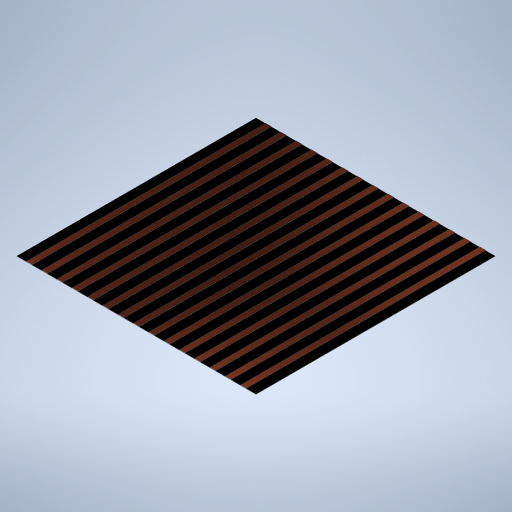
# Autodesk Inventor part: Sensor Grid Rows-Collumns
Saved by Autodesk Inventor 2023 (Build 270158000, 158)
## iProperties
Created: 2022-11-30
Part Number: Sensor Grid Rows-Collumns
Material: Generic
Document SubType Name: Modeling
Designer: dylan
Density: 1 g/cm^3
Appearance: Default
Author: dylan
Autodesk Inventor part; units mm, degrees
ref_plane "YZ Plane" through (0, 0, 0) normal (1, 0, 0) x (0, 1, 0)
ref_plane "XZ Plane" through (0, 0, 0) normal (0, 1, 0) x (-1, 0, 0)
ref_plane "XY Plane" through (0, 0, 0) normal (0, 0, 1) x (1, 0, 0)
sketch "Sketch1" plane through (0, 0, 0) normal (0, 1, 0) x (-1, 0, 0)
  line L0 (0, 0) -> (800, 0)
  line L1 (800, 0) -> (800, -800)
  line L2 (800, -800) -> (0, -800)
  line L3 (0, -800) -> (0, 0)
  line L4 (0, 0) -> (32.14, 0)
  line L5 (32.14, 0) -> (32.14, -800)
  line L6 (32.14, -800) -> (0, -800)
  line L7 (0, -800) -> (0, 0)
  line L8 (32.14, 0) -> (51.19, 0)
  line L9 (51.19, 0) -> (51.19, -800)
  line L10 (51.19, -800) -> (32.14, -800)
  line L11 (32.14, -800) -> (32.14, 0)
  line L12 (51.19, 0) -> (83.33, 0)
  line L13 (83.33, 0) -> (83.33, -800)
  line L14 (83.33, -800) -> (51.19, -800)
  line L15 (51.19, -800) -> (51.19, 0)
  line L16 (83.33, 0) -> (102.38, 0)
  line L17 (102.38, 0) -> (102.38, -800)
  line L18 (102.38, -800) -> (83.33, -800)
  line L19 (83.33, -800) -> (83.33, 0)
  line L20 (102.38, 0) -> (134.52, 0)
  line L21 (134.52, 0) -> (134.52, -800)
  line L22 (134.52, -800) -> (102.38, -800)
  line L23 (102.38, -800) -> (102.38, 0)
  line L24 (134.52, 0) -> (153.57, 0)
  line L25 (153.57, 0) -> (153.57, -800)
  line L26 (153.57, -800) -> (134.52, -800)
  line L27 (134.52, -800) -> (134.52, 0)
  line L28 (153.57, 0) -> (185.71, 0)
  line L29 (185.71, 0) -> (185.71, -800)
  line L30 (185.71, -800) -> (153.57, -800)
  line L31 (153.57, -800) -> (153.57, 0)
  line L32 (185.71, 0) -> (204.76, 0)
  line L33 (204.76, 0) -> (204.76, -800)
  line L34 (204.76, -800) -> (185.71, -800)
  line L35 (185.71, -800) -> (185.71, 0)
  line L36 (204.76, 0) -> (236.9, 0)
  line L37 (236.9, 0) -> (236.9, -800)
  line L38 (236.9, -800) -> (204.76, -800)
  line L39 (204.76, -800) -> (204.76, 0)
  line L40 (236.9, 0) -> (255.95, 0)
  line L41 (255.95, 0) -> (255.95, -800)
  line L42 (255.95, -800) -> (236.9, -800)
  line L43 (236.9, -800) -> (236.9, 0)
  line L44 (255.95, 0) -> (288.09, 0)
  line L45 (288.09, 0) -> (288.09, -800)
  line L46 (288.09, -800) -> (255.95, -800)
  line L47 (255.95, -800) -> (255.95, 0)
  line L48 (288.09, 0) -> (307.14, 0)
  line L49 (307.14, 0) -> (307.14, -800)
  line L50 (307.14, -800) -> (288.09, -800)
  line L51 (288.09, -800) -> (288.09, 0)
  line L52 (307.14, 0) -> (339.28, 0)
  line L53 (339.28, 0) -> (339.28, -800)
  line L54 (339.28, -800) -> (307.14, -800)
  line L55 (307.14, -800) -> (307.14, 0)
  line L56 (339.28, 0) -> (358.33, 0)
  line L57 (358.33, 0) -> (358.33, -800)
  line L58 (358.33, -800) -> (339.28, -800)
  line L59 (339.28, -800) -> (339.28, 0)
  line L60 (358.33, 0) -> (390.47, 0)
  line L61 (390.47, 0) -> (390.47, -800)
  line L62 (390.47, -800) -> (358.33, -800)
  line L63 (358.33, -800) -> (358.33, 0)
  line L64 (390.47, 0) -> (409.52, 0)
  line L65 (409.52, 0) -> (409.52, -800)
  line L66 (409.52, -800) -> (390.47, -800)
  line L67 (390.47, -800) -> (390.47, 0)
  line L68 (409.52, 0) -> (441.66, 0)
  line L69 (441.66, 0) -> (441.66, -800)
  line L70 (441.66, -800) -> (409.52, -800)
  line L71 (409.52, -800) -> (409.52, 0)
  line L72 (441.66, 0) -> (460.71, 0)
  line L73 (460.71, 0) -> (460.71, -800)
  line L74 (460.71, -800) -> (441.66, -800)
  line L75 (441.66, -800) -> (441.66, 0)
  line L76 (460.71, 0) -> (492.85, 0)
  line L77 (492.85, 0) -> (492.85, -800)
  line L78 (492.85, -800) -> (460.71, -800)
  line L79 (460.71, -800) -> (460.71, 0)
  line L80 (492.85, 0) -> (511.9, 0)
  line L81 (511.9, 0) -> (511.9, -800)
  line L82 (511.9, -800) -> (492.85, -800)
  line L83 (492.85, -800) -> (492.85, 0)
  line L84 (511.9, 0) -> (544.04, 0)
  line L85 (544.04, 0) -> (544.04, -800)
  line L86 (544.04, -800) -> (511.9, -800)
  line L87 (511.9, -800) -> (511.9, 0)
  line L88 (544.04, 0) -> (563.09, 0)
  line L89 (563.09, 0) -> (563.09, -800)
  line L90 (563.09, -800) -> (544.04, -800)
  line L91 (544.04, -800) -> (544.04, 0)
  line L92 (563.09, 0) -> (595.23, 0)
  line L93 (595.23, 0) -> (595.23, -800)
  line L94 (595.23, -800) -> (563.09, -800)
  line L95 (563.09, -800) -> (563.09, 0)
  line L96 (595.23, 0) -> (614.28, 0)
  line L97 (614.28, 0) -> (614.28, -800)
  line L98 (614.28, -800) -> (595.23, -800)
  line L99 (595.23, -800) -> (595.23, 0)
  line L100 (614.28, 0) -> (646.42, 0)
  line L101 (646.42, 0) -> (646.42, -800)
  line L102 (646.42, -800) -> (614.28, -800)
  line L103 (614.28, -800) -> (614.28, 0)
  line L104 (646.42, 0) -> (665.47, 0)
  line L105 (665.47, 0) -> (665.47, -800)
  line L106 (665.47, -800) -> (646.42, -800)
  line L107 (646.42, -800) -> (646.42, 0)
  line L108 (665.47, 0) -> (697.61, 0)
  line L109 (697.61, 0) -> (697.61, -800)
  line L110 (697.61, -800) -> (665.47, -800)
  line L111 (665.47, -800) -> (665.47, 0)
  line L112 (697.61, 0) -> (716.66, 0)
  line L113 (716.66, 0) -> (716.66, -800)
  line L114 (716.66, -800) -> (697.61, -800)
  line L115 (697.61, -800) -> (697.61, 0)
  line L116 (716.66, 0) -> (748.8, 0)
  line L117 (748.8, 0) -> (748.8, -800)
  line L118 (748.8, -800) -> (716.66, -800)
  line L119 (716.66, -800) -> (716.66, 0)
  line L120 (748.8, 0) -> (767.85, 0)
  line L121 (767.85, 0) -> (767.85, -800)
  line L122 (767.85, -800) -> (748.8, -800)
  line L123 (748.8, -800) -> (748.8, 0)
  dimension "d0" = 800
  dimension "d1" = 800
  dimension "d2" = 32.14
  dimension "d4" = 19.05
  dimension "d6" = 32.14
  dimension "d7" = 19.05
  dimension "d8" = 32.14
  dimension "d9" = 19.05
  dimension "d10" = 32.14
  dimension "d11" = 19.05
  dimension "d12" = 32.14
  dimension "d13" = 19.05
  dimension "d14" = 32.14
  dimension "d15" = 19.05
  dimension "d16" = 32.14
  dimension "d17" = 19.05
  dimension "d18" = 32.14
  dimension "d19" = 19.05
  dimension "d20" = 32.14
  dimension "d21" = 19.05
  dimension "d22" = 32.14
  dimension "d23" = 19.05
  dimension "d24" = 32.14
  dimension "d25" = 19.05
  dimension "d26" = 32.14
  dimension "d27" = 19.05
  dimension "d28" = 32.14
  dimension "d29" = 19.05
  dimension "d30" = 32.14
  dimension "d31" = 19.05
  dimension "d32" = 32.14
  dimension "d33" = 19.05
  constraints: 244 end point, 61 parallel, 30 horizontal, 30 perpendicular, 1 vertical, 6 other
  measures "d0" distance of L1.end L3.start
  measures "d1" distance of L1.start L1.end
  measures "d2" distance of L5.end L6.end
  measures "d4" distance of L9.end L10.end
  measures "d6" distance of L13.end L14.end
  measures "d7" distance of L17.end L18.end
  measures "d8" distance of L21.end L22.end
  measures "d9" distance of L25.end L26.end
  measures "d10" distance of L29.end L30.end
  measures "d11" distance of L33.end L34.end
  measures "d12" distance of L37.end L38.end
  measures "d13" distance of L41.end L42.end
  measures "d14" distance of L45.end L46.end
  measures "d15" distance of L49.end L50.end
  measures "d16" distance of L53.end L54.end
  measures "d17" distance of L57.end L58.end
  measures "d18" distance of L61.end L62.end
  measures "d19" distance of L65.end L66.end
  measures "d20" distance of L69.end L70.end
  measures "d21" distance of L73.end L74.end
  measures "d22" distance of L77.end L78.end
  measures "d23" distance of L81.end L82.end
  measures "d24" distance of L85.end L86.end
  measures "d25" distance of L89.end L90.end
  measures "d26" distance of L93.end L94.end
  measures "d27" distance of L97.end L98.end
  measures "d28" distance of L101.end L102.end
  measures "d29" distance of L105.end L106.end
  measures "d30" distance of L109.end L110.end
  measures "d31" distance of L113.end L114.end
  measures "d32" distance of L117.end L118.end
  measures "d33" distance of L121.end L122.end
extrude "Extrusion1" add sketch "Sketch1" along normal blind 1 contours L0 L5 L2 L3 | L0 L13 L2 L9 | L0 L21 L2 L17 | L0 L29 L2 L25 | L0 L37 L2 L33 | L0 L45 L2 L41 | L0 L53 L2 L49 | L0 L61 L2 L57 | L0 L69 L2 L65 | L0 L77 L2 L73 | L0 L85 L2 L81 | L0 L93 L2 L89 | L0 L101 L2 L97 | L0 L109 L2 L105 | L0 L117 L2 L113 | L0 L1 L2 L121
extrude "Extrusion2" add sketch "Sketch1" along normal blind 2 contours L0 L9 L2 L5 | L0 L17 L2 L13 | L0 L25 L2 L21 | L0 L33 L2 L29 | L0 L41 L2 L37 | L0 L49 L2 L45 | L0 L57 L2 L53 | L0 L65 L2 L61 | L0 L73 L2 L69 | L0 L81 L2 L77 | L0 L89 L2 L85 | L0 L97 L2 L93 | L0 L105 L2 L101 | L0 L113 L2 L109 | L0 L121 L2 L117
